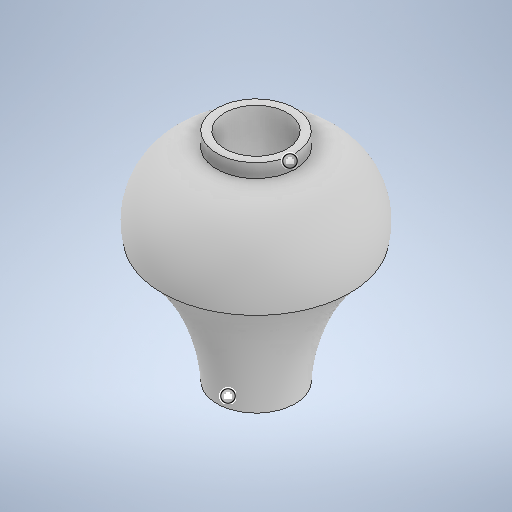
# Autodesk Inventor part: Water Sensor Bouy
Saved by Autodesk Inventor 2025 (Build 290162000, 162)
## iProperties
Created: 2024-06-17
Part Number: Water Sensor Bouy
Material: Generic
Document SubType Name: Modeling
Designer: track
Density: 1 g/cm^3
Appearance: Default
Mass: 885.051 g
Surface Area: 1766.64 cm^2
Volume: 885.051 cm^3
Author: track
## iProperties of the stored document Water Sensor Bouy_3DPrint.ipt
Created: 2024-06-17
Part Number: Water Sensor Bouy_3DPrint
Material: Generic
Document SubType Name: Modeling
Designer: track
Density: 1 g/cm^3
Appearance: Default
Author: track
Autodesk Inventor part; units mm, degrees
ref_plane "Work Plane4" through (55.0851, 96.0393, 0) normal (0.3608, 0.9326, 0) x (-0.9326, 0.3608, 0)
ref_plane "YZ Plane" through (0, 0, 0) normal (1, 0, 0) x (0, 1, 0)
ref_plane "XZ Plane" through (0, 0, 0) normal (0, 1, 0) x (-1, 0, 0)
sketch "Sketch1" plane through (0, 0, 0) normal (0, 0, 1) x (1, 0, 0)
  line L0 (0, 0) -> (0, 76.2)
  line L1 (25.32, 0) -> (25.32, 165.1)
  arc A0 (76.12, 99.9869) -> (31.7961, 164.6981) centre (25.32, 112.7269) ccw
  line L2 (25.32, 0) -> (31.67, 0)
  arc A1 (76.12, 99.9869) -> (31.67, 0) centre (183.8709, -7.7884) ccw
  line L3 (27.32, 163.0603) -> (27.32, 2)
  line L4 (27.32, 2) -> (29.7814, 2)
  arc A2 (74.3101, 101.0041) -> (29.7814, 2) centre (183.8709, -7.7884) ccw
  arc A3 (74.3101, 101.0041) -> (27.32, 163.0603) centre (25.32, 112.7269) ccw
  line L5 (25.32, 175.7603) -> (25.32, 165.1)
  line L6 (25.32, 175.7603) -> (31.67, 175.7603)
  line L7 (31.67, 175.7603) -> (31.7961, 164.6981)
  point P0 (25.32, 25.4)
  dimension "d0" = 165.1
  dimension "d1" = 25.32
  dimension "d3" = 0
  dimension "d24" = 52.3732
  dimension "d159" = 6.35
  dimension "d160" = 152.4
  dimension "d161" = 2
  dimension "d162" = 50.8
  dimension "d165" = 6.35
  dimension "d34" = 60
  dimension "d35" = 12.7
  constraints: 16 end point, 8 point on circle, 4 centre point, 2 horizontal, 2 point on line, 2 vertical, 2 other
  measures "d0" distance of L1.start L1.end
  measures "d1" distance between parallel lines of L1 L0
  measures "d3" vertical distance of L0.start L1.start
  measures "d24" radius of A0
  measures "d159" distance of L1.start L2.end
  measures "d160" radius of A1
  measures "d161" radial gap between concentric circles of A0 A3
  measures "d162" distance from line of L1 A0.start
  measures "d165" distance of L5.start L6.end
revolve "Revolution1" add sketch "Sketch1" angle 360 about axis through (0, 0, 0) along (0, 1, 0) contours L1 L5 L6 L7 A0 A1 L2 | A3 A2 L4 L3
body "Solid1"
